Autodesk Inventor part; units mm, degrees
(part 2 of 2)
  spline S325 degree 2 poles (-2.5873, -27.7967) (-2.5873, -27.5088) (-2.9583, -27.0081) (-3.2851, -26.8732) knots 0 0 0 1 2 2 2
  spline S326 degree 2 poles (-3.2851, -26.8732) (-3.5393, -26.7669) (-3.9803, -26.7513) knots 0 0 0 1 1 1
  line L146 (-3.9803, -26.7513) -> (-3.3707, -25.5192)
  line L147 (-3.3707, -25.5192) -> (-2.232, -25.5192)
  line L148 (-1.433, -25.5192) -> (0.2686, -25.5192)
  line L149 (0.2686, -25.5192) -> (0.2686, -25.6074)
  line L150 (0.2686, -25.6074) -> (-0.7897, -28.759)
  line L151 (-0.7897, -28.759) -> (-1.0517, -28.759)
  line L152 (-1.0517, -28.759) -> (-0.1023, -25.9005)
  line L153 (-0.1023, -25.9005) -> (-0.9765, -25.9005)
  spline S327 degree 2 poles (-0.9765, -25.9005) (-1.2411, -25.9005) (-1.3526, -25.9628) knots 0 0 0 1 1 1
  spline S328 degree 2 poles (-1.3526, -25.9628) (-1.5498, -26.0717) (-1.6691, -26.2974) knots 0 0 0 1 1 1
  line L154 (-1.6691, -26.2974) -> (-1.7365, -26.2714)
  line L155 (-1.7365, -26.2714) -> (-1.433, -25.5192)
  spline S329 degree 2 poles (0.6577, -27.1248) (0.6577, -26.5827) (0.9845, -25.7993) (1.2569, -25.6074) knots 0 0 0 1 2 2 2
  spline S330 degree 2 poles (1.2569, -25.6074) (1.467, -25.4543) (1.6927, -25.4543) knots 0 0 0 1 1 1
  spline S331 degree 2 poles (1.6927, -25.4543) (2.0584, -25.4543) (2.3489, -25.8253) knots 0 0 0 1 1 1
  spline S332 degree 2 poles (2.3489, -25.8253) (2.7121, -26.287) (2.7121, -27.0756) knots 0 0 0 1 1 1
  spline S333 degree 2 poles (2.7121, -27.0756) (2.7121, -27.6281) (2.393, -28.4011) (1.9002, -28.7487) (1.6693, -28.7487) knots 0 0 0 1 2 3 3 3
  spline S334 degree 2 poles (1.6693, -28.7487) (1.2154, -28.7487) (0.9119, -28.2117) knots 0 0 0 1 1 1
  spline S335 degree 2 poles (0.9119, -28.2117) (0.6577, -27.7604) (0.6577, -27.1248) knots 0 0 0 1 1 1
  spline S336 degree 2 poles (1.1168, -27.1845) (1.1168, -27.8382) (1.2776, -28.2532) knots 0 0 0 1 1 1
  spline S337 degree 2 poles (1.2776, -28.2532) (1.4125, -28.6008) (1.6771, -28.6008) knots 0 0 0 1 1 1
  spline S338 degree 2 poles (1.6771, -28.6008) (1.8042, -28.6008) (2.074, -28.3751) (2.144, -28.108) knots 0 0 0 1 2 2 2
  spline S339 degree 2 poles (2.144, -28.108) (2.253, -27.7059) (2.253, -26.9744) knots 0 0 0 1 1 1
  spline S340 degree 2 poles (2.253, -26.9744) (2.253, -26.4297) (2.1414, -26.0691) knots 0 0 0 1 1 1
  spline S341 degree 2 poles (2.1414, -26.0691) (2.0558, -25.7993) (1.9235, -25.6878) knots 0 0 0 1 1 1
  spline S342 degree 2 poles (1.9235, -25.6878) (1.8276, -25.61) (1.6901, -25.61) knots 0 0 0 1 1 1
  spline S343 degree 2 poles (1.6901, -25.61) (1.5318, -25.61) (1.4073, -25.7526) knots 0 0 0 1 1 1
  spline S344 degree 2 poles (1.4073, -25.7526) (1.2387, -25.9472) (1.1168, -26.7798) (1.1168, -27.1845) knots 0 0 0 1 2 2 2
  spline S345 degree 2 poles (3.0571, -27.1248) (3.0571, -26.5827) (3.3839, -25.7993) (3.6563, -25.6074) knots 0 0 0 1 2 2 2
  spline S346 degree 2 poles (3.6563, -25.6074) (3.8664, -25.4543) (4.0921, -25.4543) knots 0 0 0 1 1 1
  spline S347 degree 2 poles (4.0921, -25.4543) (4.4578, -25.4543) (4.7484, -25.8253) knots 0 0 0 1 1 1
  spline S348 degree 2 poles (4.7484, -25.8253) (5.1115, -26.287) (5.1115, -27.0756) knots 0 0 0 1 1 1
  spline S349 degree 2 poles (5.1115, -27.0756) (5.1115, -27.6281) (4.7925, -28.4011) (4.2996, -28.7487) (4.0687, -28.7487) knots 0 0 0 1 2 3 3 3
  spline S350 degree 2 poles (4.0687, -28.7487) (3.6148, -28.7487) (3.3113, -28.2117) knots 0 0 0 1 1 1
  spline S351 degree 2 poles (3.3113, -28.2117) (3.0571, -27.7604) (3.0571, -27.1248) knots 0 0 0 1 1 1
  spline S352 degree 2 poles (3.5162, -27.1845) (3.5162, -27.8382) (3.677, -28.2532) knots 0 0 0 1 1 1
  spline S353 degree 2 poles (3.677, -28.2532) (3.8119, -28.6008) (4.0765, -28.6008) knots 0 0 0 1 1 1
  spline S354 degree 2 poles (4.0765, -28.6008) (4.2036, -28.6008) (4.4734, -28.3751) (4.5434, -28.108) knots 0 0 0 1 2 2 2
  spline S355 degree 2 poles (4.5434, -28.108) (4.6524, -27.7059) (4.6524, -26.9744) knots 0 0 0 1 1 1
  spline S356 degree 2 poles (4.6524, -26.9744) (4.6524, -26.4297) (4.5408, -26.0691) knots 0 0 0 1 1 1
  spline S357 degree 2 poles (4.5408, -26.0691) (4.4552, -25.7993) (4.3229, -25.6878) knots 0 0 0 1 1 1
  spline S358 degree 2 poles (4.3229, -25.6878) (4.227, -25.61) (4.0895, -25.61) knots 0 0 0 1 1 1
  spline S359 degree 2 poles (4.0895, -25.61) (3.9313, -25.61) (3.8067, -25.7526) knots 0 0 0 1 1 1
  spline S360 degree 2 poles (3.8067, -25.7526) (3.6381, -25.9472) (3.5162, -26.7798) (3.5162, -27.1845) knots 0 0 0 1 2 2 2
  spline S361 degree 2 poles (5.4565, -27.1248) (5.4565, -26.5827) (5.7833, -25.7993) (6.0557, -25.6074) knots 0 0 0 1 2 2 2
  spline S362 degree 2 poles (6.0557, -25.6074) (6.2658, -25.4543) (6.4915, -25.4543) knots 0 0 0 1 1 1
  spline S363 degree 2 poles (6.4915, -25.4543) (6.8572, -25.4543) (7.1478, -25.8253) knots 0 0 0 1 1 1
  spline S364 degree 2 poles (7.1478, -25.8253) (7.5109, -26.287) (7.5109, -27.0756) knots 0 0 0 1 1 1
  spline S365 degree 2 poles (7.5109, -27.0756) (7.5109, -27.6281) (7.1919, -28.4011) (6.699, -28.7487) (6.4681, -28.7487) knots 0 0 0 1 2 3 3 3
  spline S366 degree 2 poles (6.4681, -28.7487) (6.0142, -28.7487) (5.7107, -28.2117) knots 0 0 0 1 1 1
  spline S367 degree 2 poles (5.7107, -28.2117) (5.4565, -27.7604) (5.4565, -27.1248) knots 0 0 0 1 1 1
  spline S368 degree 2 poles (5.9156, -27.1845) (5.9156, -27.8382) (6.0765, -28.2532) knots 0 0 0 1 1 1
  spline S369 degree 2 poles (6.0765, -28.2532) (6.2113, -28.6008) (6.4759, -28.6008) knots 0 0 0 1 1 1
  spline S370 degree 2 poles (6.4759, -28.6008) (6.603, -28.6008) (6.8728, -28.3751) (6.9428, -28.108) knots 0 0 0 1 2 2 2
  spline S371 degree 2 poles (6.9428, -28.108) (7.0518, -27.7059) (7.0518, -26.9744) knots 0 0 0 1 1 1
  spline S372 degree 2 poles (7.0518, -26.9744) (7.0518, -26.4297) (6.9402, -26.0691) knots 0 0 0 1 1 1
  spline S373 degree 2 poles (6.9402, -26.0691) (6.8546, -25.7993) (6.7224, -25.6878) knots 0 0 0 1 1 1
  spline S374 degree 2 poles (6.7224, -25.6878) (6.6264, -25.61) (6.4889, -25.61) knots 0 0 0 1 1 1
  spline S375 degree 2 poles (6.4889, -25.61) (6.3307, -25.61) (6.2062, -25.7526) knots 0 0 0 1 1 1
  spline S376 degree 2 poles (6.2062, -25.7526) (6.0375, -25.9472) (5.9156, -26.7798) (5.9156, -27.1845) knots 0 0 0 1 2 2 2
  line L156 (8.2424, -25.8305) -> (9.0154, -25.4543)
  line L157 (9.0154, -25.4543) -> (9.0932, -25.4543)
  line L158 (9.0932, -25.4543) -> (9.0932, -28.1339)
  spline S377 degree 2 poles (9.0932, -28.1339) (9.0932, -28.4011) (9.1373, -28.5334) (9.2774, -28.6034) (9.4927, -28.6086) knots 0 0 0 1 2 3 3 3
  line L159 (9.4927, -28.6086) -> (9.4927, -28.6942)
  line L160 (9.4927, -28.6942) -> (8.2995, -28.6942)
  line L161 (8.2995, -28.6942) -> (8.2995, -28.6086)
  spline S378 degree 2 poles (8.2995, -28.6086) (8.5252, -28.6034) (8.6548, -28.536) (8.7067, -28.4218) (8.7067, -28.1339) knots 0 0 0 1 2 3 3 3
  line L162 (8.7067, -28.1339) -> (8.7067, -26.4219)
  spline S379 degree 2 poles (8.7067, -26.4219) (8.7067, -26.0743) (8.6834, -25.9757) knots 0 0 0 1 1 1
  spline S380 degree 2 poles (8.6834, -25.9757) (8.6678, -25.9005) (8.5796, -25.8305) (8.52, -25.8305) knots 0 0 0 1 2 2 2
  spline S381 degree 2 poles (8.52, -25.8305) (8.4318, -25.8305) (8.2787, -25.9031) knots 0 0 0 1 1 1
  line L163 (8.2787, -25.9031) -> (8.2424, -25.8305)
  line L164 (-11.5767, -33.1063) -> (-11.7998, -33.7159)
  line L165 (-11.7998, -33.7159) -> (-13.6726, -33.7159)
  line L166 (-13.6726, -33.7159) -> (-13.6726, -33.6303)
  spline S382 degree 2 poles (-13.6726, -33.6303) (-12.8451, -32.8755) (-12.1707, -31.9209) (-12.1707, -31.524) knots 0 0 0 1 2 2 2
  spline S383 degree 2 poles (-12.1707, -31.524) (-12.1707, -31.2231) (-12.5416, -30.834) (-12.7985, -30.834) knots 0 0 0 1 2 2 2
  spline S384 degree 2 poles (-12.7985, -30.834) (-13.0345, -30.834) (-13.4054, -31.109) (-13.4962, -31.3736) knots 0 0 0 1 2 2 2
  line L167 (-13.4962, -31.3736) -> (-13.5818, -31.3736)
  spline S385 degree 2 poles (-13.5818, -31.3736) (-13.5222, -30.9404) (-13.0397, -30.4761) (-12.6765, -30.4761) knots 0 0 0 1 2 2 2
  spline S386 degree 2 poles (-12.6765, -30.4761) (-12.29, -30.4761) (-11.7712, -30.9715) (-11.7712, -31.3087) knots 0 0 0 1 2 2 2
  spline S387 degree 2 poles (-11.7712, -31.3087) (-11.7712, -31.55) (-11.8828, -31.7912) knots 0 0 0 1 1 1
  spline S388 degree 2 poles (-11.8828, -31.7912) (-12.0566, -32.1699) (-12.4457, -32.5953) knots 0 0 0 1 1 1
  spline S389 degree 2 poles (-12.4457, -32.5953) (-13.0293, -33.2308) (-13.1746, -33.3631) knots 0 0 0 1 1 1
  line L168 (-13.1746, -33.3631) -> (-12.3445, -33.3631)
  spline S390 degree 2 poles (-12.3445, -33.3631) (-12.0903, -33.3631) (-11.888, -33.3268) (-11.7246, -33.2101) (-11.6623, -33.1063) knots 0 0 0 1 2 3 3 3
  line L169 (-11.6623, -33.1063) -> (-11.5767, -33.1063)
  spline S391 degree 2 poles (-10.5988, -31.9624) (-10.2227, -31.5084) (-9.8803, -31.5084) knots 0 0 0 1 1 1
  spline S392 degree 2 poles (-9.8803, -31.5084) (-9.7065, -31.5084) (-9.4548, -31.6848) (-9.3796, -31.8846) knots 0 0 0 1 2 2 2
  spline S393 degree 2 poles (-9.3796, -31.8846) (-9.3277, -32.0246) (-9.3277, -32.3152) knots 0 0 0 1 1 1
  line L170 (-9.3277, -32.3152) -> (-9.3277, -33.2308)
  spline S394 degree 2 poles (-9.3277, -33.2308) (-9.3277, -33.4332) (-9.294, -33.5058) knots 0 0 0 1 1 1
  spline S395 degree 2 poles (-9.294, -33.5058) (-9.2681, -33.5655) (-9.1539, -33.6303) (-9.0009, -33.6303) knots 0 0 0 1 2 2 2
  line L171 (-9.0009, -33.6303) -> (-9.0009, -33.7159)
  line L172 (-9.0009, -33.7159) -> (-10.0644, -33.7159)
  line L173 (-10.0644, -33.7159) -> (-10.0644, -33.6303)
  line L174 (-10.0644, -33.6303) -> (-10.0203, -33.6303)
  spline S396 degree 2 poles (-10.0203, -33.6303) (-9.8699, -33.6303) (-9.7506, -33.5395) (-9.7272, -33.4513) knots 0 0 0 1 2 2 2
  spline S397 degree 2 poles (-9.7272, -33.4513) (-9.7168, -33.415) (-9.7168, -33.2308) knots 0 0 0 1 1 1
  line L175 (-9.7168, -33.2308) -> (-9.7168, -32.3541)
  spline S398 degree 2 poles (-9.7168, -32.3541) (-9.7168, -32.061) (-9.8673, -31.7964) (-10.0463, -31.7964) knots 0 0 0 1 2 2 2
  spline S399 degree 2 poles (-10.0463, -31.7964) (-10.3238, -31.7964) (-10.5988, -32.0999) knots 0 0 0 1 1 1
  line L176 (-10.5988, -32.0999) -> (-10.5988, -33.2308)
  spline S400 degree 2 poles (-10.5988, -33.2308) (-10.5988, -33.4487) (-10.5728, -33.5006) knots 0 0 0 1 1 1
  spline S401 degree 2 poles (-10.5728, -33.5006) (-10.5391, -33.568) (-10.425, -33.6303) (-10.2486, -33.6303) knots 0 0 0 1 2 2 2
  line L177 (-10.2486, -33.6303) -> (-10.2486, -33.7159)
  line L178 (-10.2486, -33.7159) -> (-11.3147, -33.7159)
  line L179 (-11.3147, -33.7159) -> (-11.3147, -33.6303)
  line L180 (-11.3147, -33.6303) -> (-11.268, -33.6303)
  spline S402 degree 2 poles (-11.268, -33.6303) (-11.102, -33.6303) (-10.9879, -33.4643) (-10.9879, -33.2308) knots 0 0 0 1 2 2 2
  line L181 (-10.9879, -33.2308) -> (-10.9879, -32.4345)
  spline S403 degree 2 poles (-10.9879, -32.4345) (-10.9879, -32.0506) (-11.0242, -31.882) (-11.0968, -31.8197) (-11.1565, -31.8197) knots 0 0 0 1 2 3 3 3
  spline S404 degree 2 poles (-11.1565, -31.8197) (-11.2213, -31.8197) (-11.3121, -31.856) knots 0 0 0 1 1 1
  line L182 (-11.3121, -31.856) -> (-11.3484, -31.7704)
  line L183 (-11.3484, -31.7704) -> (-10.6999, -31.5084)
  line L184 (-10.6999, -31.5084) -> (-10.5988, -31.5084)
  line L185 (-10.5988, -31.5084) -> (-10.5988, -31.9624)
  spline S405 degree 2 poles (-7.3148, -33.4747) (-7.4705, -33.6381) (-7.7714, -33.7808) (-7.9452, -33.7808) knots 0 0 0 1 2 2 2
  spline S406 degree 2 poles (-7.9452, -33.7808) (-8.2953, -33.7808) (-8.8193, -33.1945) (-8.8193, -32.7328) knots 0 0 0 1 2 2 2
  spline S407 degree 2 poles (-8.8193, -32.7328) (-8.8193, -32.2737) (-8.2383, -31.5084) (-7.7817, -31.5084) knots 0 0 0 1 2 2 2
  spline S408 degree 2 poles (-7.7817, -31.5084) (-7.499, -31.5084) (-7.3148, -31.69) knots 0 0 0 1 1 1
  line L186 (-7.3148, -31.69) -> (-7.3148, -31.288)
  spline S409 degree 2 poles (-7.3148, -31.288) (-7.3148, -30.9222) (-7.3511, -30.7562) (-7.4238, -30.6965) (-7.4808, -30.6965) knots 0 0 0 1 2 3 3 3
  spline S410 degree 2 poles (-7.4808, -30.6965) (-7.5405, -30.6965) (-7.6417, -30.7329) knots 0 0 0 1 1 1
  line L187 (-7.6417, -30.7329) -> (-7.6728, -30.6473)
  line L188 (-7.6728, -30.6473) -> (-7.0347, -30.3853)
  line L189 (-7.0347, -30.3853) -> (-6.9283, -30.3853)
  line L190 (-6.9283, -30.3853) -> (-6.9283, -32.8677)
  spline S411 degree 2 poles (-6.9283, -32.8677) (-6.9283, -33.2412) (-6.892, -33.4072) (-6.8168, -33.4721) (-6.7649, -33.4721) knots 0 0 0 1 2 3 3 3
  spline S412 degree 2 poles (-6.7649, -33.4721) (-6.7027, -33.4721) (-6.5963, -33.4332) knots 0 0 0 1 1 1
  line L191 (-6.5963, -33.4332) -> (-6.5704, -33.5188)
  line L192 (-6.5704, -33.5188) -> (-7.2059, -33.7808)
  line L193 (-7.2059, -33.7808) -> (-7.3148, -33.7808)
  line L194 (-7.3148, -33.7808) -> (-7.3148, -33.4747)
  line L195 (-7.3148, -33.3087) -> (-7.3148, -32.2088)
  spline S413 degree 2 poles (-7.3148, -32.2088) (-7.3278, -32.048) (-7.4705, -31.786) (-7.7013, -31.6537) (-7.8103, -31.6537) knots 0 0 0 1 2 3 3 3
  spline S414 degree 2 poles (-7.8103, -31.6537) (-8.0178, -31.6537) (-8.1786, -31.8379) knots 0 0 0 1 1 1
  spline S415 degree 2 poles (-8.1786, -31.8379) (-8.3913, -32.0817) (-8.3913, -32.5486) knots 0 0 0 1 1 1
  spline S416 degree 2 poles (-8.3913, -32.5486) (-8.3913, -33.0207) (-7.9789, -33.5239) (-7.7273, -33.5239) knots 0 0 0 1 2 2 2
  spline S417 degree 2 poles (-7.7273, -33.5239) (-7.5146, -33.5239) (-7.3148, -33.3087) knots 0 0 0 1 1 1
  line L196 (-3.1749, -30.4683) -> (-3.1749, -31.5655)
  line L197 (-3.1749, -31.5655) -> (-3.2605, -31.5655)
  spline S418 degree 2 poles (-3.2605, -31.5655) (-3.302, -31.2491) (-3.5225, -30.8755) (-3.9245, -30.655) (-4.1424, -30.655) knots 0 0 0 1 2 3 3 3
  spline S419 degree 2 poles (-4.1424, -30.655) (-4.3863, -30.655) (-4.7053, -30.9533) (-4.7053, -31.1427) knots 0 0 0 1 2 2 2
  spline S420 degree 2 poles (-4.7053, -31.1427) (-4.7053, -31.288) (-4.6041, -31.4073) knots 0 0 0 1 1 1
  spline S421 degree 2 poles (-4.6041, -31.4073) (-4.4589, -31.5837) (-3.9116, -31.8768) knots 0 0 0 1 1 1
  spline S422 degree 2 poles (-3.9116, -31.8768) (-3.468, -32.1154) (-3.1412, -32.3696) (-2.9648, -32.7172) (-2.9648, -32.9066) knots 0 0 0 1 2 3 3 3
  spline S423 degree 2 poles (-2.9648, -32.9066) (-2.9648, -33.2671) (-3.5251, -33.7885) (-3.966, -33.7885) knots 0 0 0 1 2 2 2
  spline S424 degree 2 poles (-3.966, -33.7885) (-4.1035, -33.7885) (-4.2254, -33.7678) knots 0 0 0 1 1 1
  spline S425 degree 2 poles (-4.2254, -33.7678) (-4.2981, -33.7548) (-4.7546, -33.607) (-4.8169, -33.607) knots 0 0 0 1 2 2 2
  spline S426 degree 2 poles (-4.8169, -33.607) (-4.8739, -33.607) (-4.944, -33.677) (-4.9595, -33.7885) knots 0 0 0 1 2 2 2
  line L198 (-4.9595, -33.7885) -> (-5.0451, -33.7885)
  line L199 (-5.0451, -33.7885) -> (-5.0451, -32.6991)
  line L200 (-5.0451, -32.6991) -> (-4.9595, -32.6991)
  spline S427 degree 2 poles (-4.9595, -32.6991) (-4.8999, -33.0415) (-4.6923, -33.3813) (-4.2669, -33.607) (-4.0153, -33.607) knots 0 0 0 1 2 3 3 3
  spline S428 degree 2 poles (-4.0153, -33.607) (-3.7222, -33.607) (-3.3824, -33.2983) (-3.3824, -33.0856) knots 0 0 0 1 2 2 2
  spline S429 degree 2 poles (-3.3824, -33.0856) (-3.3824, -32.9688) (-3.5121, -32.7302) (-3.647, -32.6264) knots 0 0 0 1 2 2 2
  spline S430 degree 2 poles (-3.647, -32.6264) (-3.7378, -32.5564) (-4.5549, -32.0999) (-4.8999, -31.8275) (-5.0788, -31.5007) (-5.0788, -31.3035) knots 0 0 0 1 2 3 4 4 4
  spline S431 degree 2 poles (-5.0788, -31.3035) (-5.0788, -30.9611) (-4.5523, -30.4683) (-4.145, -30.4683) knots 0 0 0 1 2 2 2
  spline S432 degree 2 poles (-4.145, -30.4683) (-3.8934, -30.4683) (-3.6081, -30.5928) knots 0 0 0 1 1 1
  spline S433 degree 2 poles (-3.6081, -30.5928) (-3.4758, -30.6498) (-3.4213, -30.6498) knots 0 0 0 1 1 1
  spline S434 degree 2 poles (-3.4213, -30.6498) (-3.3616, -30.6498) (-3.2838, -30.5772) (-3.2605, -30.4683) knots 0 0 0 1 2 2 2
  line L201 (-3.2605, -30.4683) -> (-3.1749, -30.4683)
  spline S435 degree 2 poles (-2.2021, -32.38) (-2.2047, -32.8573) (-1.9713, -33.1271) knots 0 0 0 1 1 1
  spline S436 degree 2 poles (-1.9713, -33.1271) (-1.7352, -33.3994) (-1.4188, -33.3994) knots 0 0 0 1 1 1
  spline S437 degree 2 poles (-1.4188, -33.3994) (-1.2087, -33.3994) (-0.8974, -33.1686) (-0.791, -32.8858) knots 0 0 0 1 2 2 2
  line L202 (-0.791, -32.8858) -> (-0.7184, -32.9325)
  spline S438 degree 2 poles (-0.7184, -32.9325) (-0.7677, -33.2542) (-1.2398, -33.7808) (-1.5978, -33.7808) knots 0 0 0 1 2 2 2
  spline S439 degree 2 poles (-1.5978, -33.7808) (-1.9843, -33.7808) (-2.5342, -33.179) (-2.5342, -32.6731) knots 0 0 0 1 2 2 2
  spline S440 degree 2 poles (-2.5342, -32.6731) (-2.5342, -32.1232) (-1.9687, -31.5084) (-1.5433, -31.5084) knots 0 0 0 1 2 2 2
  spline S441 degree 2 poles (-1.5433, -31.5084) (-1.1827, -31.5084) (-0.7184, -31.9831) (-0.7184, -32.38) knots 0 0 0 1 2 2 2
  line L203 (-0.7184, -32.38) -> (-2.2021, -32.38)
  line L204 (-2.2021, -32.2451) -> (-1.2061, -32.2451)
  spline S442 degree 2 poles (-1.2061, -32.2451) (-1.219, -32.0402) (-1.2554, -31.9546) knots 0 0 0 1 1 1
  spline S443 degree 2 poles (-1.2554, -31.9546) (-1.315, -31.8249) (-1.5459, -31.6745) (-1.673, -31.6745) knots 0 0 0 1 2 2 2
  spline S444 degree 2 poles (-1.673, -31.6745) (-1.8675, -31.6745) (-2.1762, -31.9754) (-2.2021, -32.2451) knots 0 0 0 1 2 2 2
  line L205 (-0.5887, -31.7834) -> (0.0728, -31.5162)
  line L206 (0.0728, -31.5162) -> (0.1609, -31.5162)
  line L207 (0.1609, -31.5162) -> (0.1609, -32.0195)
  spline S445 degree 2 poles (0.1609, -32.0195) (0.327, -31.7367) (0.6616, -31.5084) (0.8457, -31.5084) knots 0 0 0 1 2 2 2
  spline S446 degree 2 poles (0.8457, -31.5084) (1.17, -31.5084) (1.3853, -31.7601) knots 0 0 0 1 1 1
  spline S447 degree 2 poles (1.3853, -31.7601) (1.6499, -32.0713) (1.6499, -32.5668) knots 0 0 0 1 1 1
  spline S448 degree 2 poles (1.6499, -32.5668) (1.6499, -33.1219) (1.3308, -33.4824) knots 0 0 0 1 1 1
  spline S449 degree 2 poles (1.3308, -33.4824) (1.0688, -33.7808) (0.672, -33.7808) knots 0 0 0 1 1 1
  spline S450 degree 2 poles (0.672, -33.7808) (0.4982, -33.7808) (0.3711, -33.7315) knots 0 0 0 1 1 1
  spline S451 degree 2 poles (0.3711, -33.7315) (0.2777, -33.6977) (0.1609, -33.5914) knots 0 0 0 1 1 1
  line L208 (0.1609, -33.5914) -> (0.1609, -34.2451)
  spline S452 degree 2 poles (0.1609, -34.2451) (0.1609, -34.4656) (0.2154, -34.5849) (0.3477, -34.6549) (0.5241, -34.6549) knots 0 0 0 1 2 3 3 3
  line L209 (0.5241, -34.6549) -> (0.5241, -34.7405)
  line L210 (0.5241, -34.7405) -> (-0.6017, -34.7405)
  line L211 (-0.6017, -34.7405) -> (-0.6017, -34.6549)
  line L212 (-0.6017, -34.6549) -> (-0.542, -34.6549)
  spline S453 degree 2 poles (-0.542, -34.6549) (-0.4149, -34.6575) (-0.3215, -34.6056) knots 0 0 0 1 1 1
  spline S454 degree 2 poles (-0.3215, -34.6056) (-0.2774, -34.5797) (-0.2281, -34.4656) (-0.2281, -34.2295) knots 0 0 0 1 2 2 2
  line L213 (-0.2281, -34.2295) -> (-0.2281, -32.2036)
  spline S455 degree 2 poles (-0.2281, -32.2036) (-0.2281, -31.9935) (-0.2645, -31.882) (-0.3475, -31.8249) (-0.4175, -31.8249) knots 0 0 0 1 2 3 3 3
  spline S456 degree 2 poles (-0.4175, -31.8249) (-0.4746, -31.8249) (-0.5602, -31.8586) knots 0 0 0 1 1 1
  line L214 (-0.5602, -31.8586) -> (-0.5887, -31.7834)
  line L215 (0.1609, -32.1569) -> (0.1609, -32.9585)
  spline S457 degree 2 poles (0.1609, -32.9585) (0.1609, -33.2179) (0.1817, -33.2983) knots 0 0 0 1 1 1
  spline S458 degree 2 poles (0.1817, -33.2983) (0.2154, -33.4358) (0.4696, -33.6407) (0.6642, -33.6407) knots 0 0 0 1 2 2 2
  spline S459 degree 2 poles (0.6642, -33.6407) (0.8976, -33.6407) (1.0429, -33.4591) knots 0 0 0 1 1 1
  spline S460 degree 2 poles (1.0429, -33.4591) (1.2322, -33.2205) (1.2322, -32.7873) knots 0 0 0 1 1 1
  spline S461 degree 2 poles (1.2322, -32.7873) (1.2322, -32.2944) (1.0169, -32.0298) knots 0 0 0 1 1 1
  spline S462 degree 2 poles (1.0169, -32.0298) (0.8665, -31.8483) (0.6616, -31.8483) knots 0 0 0 1 1 1
  spline S463 degree 2 poles (0.6616, -31.8483) (0.55, -31.8483) (0.4385, -31.9053) knots 0 0 0 1 1 1
  spline S464 degree 2 poles (0.4385, -31.9053) (0.3555, -31.9468) (0.1609, -32.1569) knots 0 0 0 1 1 1
  line L216 (2.5915, -30.8651) -> (2.5915, -31.5707)
  line L217 (2.5915, -31.5707) -> (3.0921, -31.5707)
  line L218 (3.0921, -31.5707) -> (3.0921, -31.7341)
  line L219 (3.0921, -31.7341) -> (2.5915, -31.7341)
  line L220 (2.5915, -31.7341) -> (2.5915, -33.1271)
  spline S465 degree 2 poles (2.5915, -33.1271) (2.5915, -33.3346) (2.7108, -33.4799) (2.8042, -33.4799) knots 0 0 0 1 2 2 2
  spline S466 degree 2 poles (2.8042, -33.4799) (2.882, -33.4799) (3.0299, -33.3839) (3.0688, -33.2905) knots 0 0 0 1 2 2 2
  line L221 (3.0688, -33.2905) -> (3.1596, -33.2905)
  spline S467 degree 2 poles (3.1596, -33.2905) (3.0765, -33.5214) (2.7757, -33.7522) (2.6174, -33.7522) knots 0 0 0 1 2 2 2
  spline S468 degree 2 poles (2.6174, -33.7522) (2.5085, -33.7522) (2.301, -33.6329) (2.2024, -33.4098) (2.2024, -33.179) knots 0 0 0 1 2 3 3 3
  line L222 (2.2024, -33.179) -> (2.2024, -31.7341)
  line L223 (2.2024, -31.7341) -> (1.8626, -31.7341)
  line L224 (1.8626, -31.7341) -> (1.8626, -31.6563)
  spline S469 degree 2 poles (1.8626, -31.6563) (1.9923, -31.6044) (2.262, -31.3606) (2.3684, -31.192) knots 0 0 0 1 2 2 2
  spline S470 degree 2 poles (2.3684, -31.192) (2.4229, -31.1012) (2.5188, -30.8651) knots 0 0 0 1 1 1
  line L225 (2.5188, -30.8651) -> (2.5915, -30.8651)
  line L226 (6.5473, -33.1063) -> (6.3242, -33.7159)
  line L227 (6.3242, -33.7159) -> (4.4513, -33.7159)
  line L228 (4.4513, -33.7159) -> (4.4513, -33.6303)
  spline S471 degree 2 poles (4.4513, -33.6303) (5.2788, -32.8755) (5.9532, -31.9209) (5.9532, -31.524) knots 0 0 0 1 2 2 2
  spline S472 degree 2 poles (5.9532, -31.524) (5.9532, -31.2231) (5.5823, -30.834) (5.3255, -30.834) knots 0 0 0 1 2 2 2
  spline S473 degree 2 poles (5.3255, -30.834) (5.0895, -30.834) (4.7185, -31.109) (4.6277, -31.3736) knots 0 0 0 1 2 2 2
  line L229 (4.6277, -31.3736) -> (4.5421, -31.3736)
  spline S474 degree 2 poles (4.5421, -31.3736) (4.6018, -30.9404) (5.0843, -30.4761) (5.4474, -30.4761) knots 0 0 0 1 2 2 2
  spline S475 degree 2 poles (5.4474, -30.4761) (5.8339, -30.4761) (6.3527, -30.9715) (6.3527, -31.3087) knots 0 0 0 1 2 2 2
  spline S476 degree 2 poles (6.3527, -31.3087) (6.3527, -31.55) (6.2412, -31.7912) knots 0 0 0 1 1 1
  spline S477 degree 2 poles (6.2412, -31.7912) (6.0674, -32.1699) (5.6783, -32.5953) knots 0 0 0 1 1 1
  spline S478 degree 2 poles (5.6783, -32.5953) (5.0946, -33.2308) (4.9494, -33.3631) knots 0 0 0 1 1 1
  line L230 (4.9494, -33.3631) -> (5.7794, -33.3631)
  spline S479 degree 2 poles (5.7794, -33.3631) (6.0337, -33.3631) (6.236, -33.3268) (6.3994, -33.2101) (6.4617, -33.1063) knots 0 0 0 1 2 3 3 3
  line L231 (6.4617, -33.1063) -> (6.5473, -33.1063)
  spline S480 degree 2 poles (6.9208, -32.1466) (6.9208, -31.6044) (7.2476, -30.821) (7.52, -30.6291) knots 0 0 0 1 2 2 2
  spline S481 degree 2 poles (7.52, -30.6291) (7.7301, -30.4761) (7.9558, -30.4761) knots 0 0 0 1 1 1
  spline S482 degree 2 poles (7.9558, -30.4761) (8.3215, -30.4761) (8.612, -30.847) knots 0 0 0 1 1 1
  spline S483 degree 2 poles (8.612, -30.847) (8.9752, -31.3087) (8.9752, -32.0973) knots 0 0 0 1 1 1
  spline S484 degree 2 poles (8.9752, -32.0973) (8.9752, -32.6498) (8.6561, -33.4228) (8.1633, -33.7704) (7.9324, -33.7704) knots 0 0 0 1 2 3 3 3
  spline S485 degree 2 poles (7.9324, -33.7704) (7.4785, -33.7704) (7.175, -33.2334) knots 0 0 0 1 1 1
  spline S486 degree 2 poles (7.175, -33.2334) (6.9208, -32.7821) (6.9208, -32.1466) knots 0 0 0 1 1 1
  spline S487 degree 2 poles (7.3799, -32.2062) (7.3799, -32.8599) (7.5407, -33.2749) knots 0 0 0 1 1 1
  spline S488 degree 2 poles (7.5407, -33.2749) (7.6756, -33.6225) (7.9402, -33.6225) knots 0 0 0 1 1 1
  spline S489 degree 2 poles (7.9402, -33.6225) (8.0673, -33.6225) (8.3371, -33.3968) (8.4071, -33.1297) knots 0 0 0 1 2 2 2
  spline S490 degree 2 poles (8.4071, -33.1297) (8.5161, -32.7276) (8.5161, -31.9961) knots 0 0 0 1 1 1
  spline S491 degree 2 poles (8.5161, -31.9961) (8.5161, -31.4514) (8.4045, -31.0908) knots 0 0 0 1 1 1
  spline S492 degree 2 poles (8.4045, -31.0908) (8.3189, -30.821) (8.1866, -30.7095) knots 0 0 0 1 1 1
  spline S493 degree 2 poles (8.1866, -30.7095) (8.0907, -30.6317) (7.9532, -30.6317) knots 0 0 0 1 1 1
  spline S494 degree 2 poles (7.9532, -30.6317) (7.795, -30.6317) (7.6704, -30.7744) knots 0 0 0 1 1 1
  spline S495 degree 2 poles (7.6704, -30.7744) (7.5018, -30.9689) (7.3799, -31.8016) (7.3799, -32.2062) knots 0 0 0 1 2 2 2
  line L232 (11.3461, -33.1063) -> (11.123, -33.7159)
  line L233 (11.123, -33.7159) -> (9.2502, -33.7159)
  line L234 (9.2502, -33.7159) -> (9.2502, -33.6303)
  spline S496 degree 2 poles (9.2502, -33.6303) (10.0776, -32.8755) (10.7521, -31.9209) (10.7521, -31.524) knots 0 0 0 1 2 2 2
  spline S497 degree 2 poles (10.7521, -31.524) (10.7521, -31.2231) (10.3811, -30.834) (10.1243, -30.834) knots 0 0 0 1 2 2 2
  spline S498 degree 2 poles (10.1243, -30.834) (9.8883, -30.834) (9.5173, -31.109) (9.4265, -31.3736) knots 0 0 0 1 2 2 2
  line L235 (9.4265, -31.3736) -> (9.3409, -31.3736)
  spline S499 degree 2 poles (9.3409, -31.3736) (9.4006, -30.9404) (9.8831, -30.4761) (10.2462, -30.4761) knots 0 0 0 1 2 2 2
  spline S500 degree 2 poles (10.2462, -30.4761) (10.6327, -30.4761) (11.1515, -30.9715) (11.1515, -31.3087) knots 0 0 0 1 2 2 2
  spline S501 degree 2 poles (11.1515, -31.3087) (11.1515, -31.55) (11.04, -31.7912) knots 0 0 0 1 1 1
  spline S502 degree 2 poles (11.04, -31.7912) (10.8662, -32.1699) (10.4771, -32.5953) knots 0 0 0 1 1 1
  spline S503 degree 2 poles (10.4771, -32.5953) (9.8935, -33.2308) (9.7482, -33.3631) knots 0 0 0 1 1 1
  line L236 (9.7482, -33.3631) -> (10.5783, -33.3631)
  spline S504 degree 2 poles (10.5783, -33.3631) (10.8325, -33.3631) (11.0348, -33.3268) (11.1982, -33.2101) (11.2605, -33.1063) knots 0 0 0 1 2 3 3 3
  line L237 (11.2605, -33.1063) -> (11.3461, -33.1063)
  line L238 (13.6288, -30.5409) -> (13.4472, -30.9378)
  line L239 (13.4472, -30.9378) -> (12.4926, -30.9378)
  line L240 (12.4926, -30.9378) -> (12.2825, -31.3632)
  spline S505 degree 2 poles (12.2825, -31.3632) (12.9024, -31.454) (13.2656, -31.8249) knots 0 0 0 1 1 1
  spline S506 degree 2 poles (13.2656, -31.8249) (13.5769, -32.144) (13.5769, -32.5746) knots 0 0 0 1 1 1
  spline S507 degree 2 poles (13.5769, -32.5746) (13.5769, -32.8236) (13.372, -33.2516) (13.0633, -33.5499) (12.8739, -33.6407) knots 0 0 0 1 2 3 3 3
  spline S508 degree 2 poles (12.8739, -33.6407) (12.6041, -33.7704) (12.3214, -33.7704) knots 0 0 0 1 1 1
  spline S509 degree 2 poles (12.3214, -33.7704) (12.0335, -33.7704) (11.7741, -33.5758) (11.7741, -33.4591) knots 0 0 0 1 2 2 2
  spline S510 degree 2 poles (11.7741, -33.4591) (11.7741, -33.3943) (11.8804, -33.2931) (11.9634, -33.2931) knots 0 0 0 1 2 2 2
  spline S511 degree 2 poles (11.9634, -33.2931) (12.0231, -33.2931) (12.1165, -33.332) (12.2254, -33.4098) knots 0 0 0 1 2 2 2
  spline S512 degree 2 poles (12.2254, -33.4098) (12.4018, -33.5291) (12.5834, -33.5317) knots 0 0 0 1 1 1
  spline S513 degree 2 poles (12.5834, -33.5317) (12.8558, -33.5317) (13.2734, -33.1167) (13.2734, -32.8184) knots 0 0 0 1 2 2 2
  spline S514 degree 2 poles (13.2734, -32.8184) (13.2734, -32.5305) (12.9024, -32.0298) (12.5756, -31.8949) knots 0 0 0 1 2 2 2
  spline S515 degree 2 poles (12.5756, -31.8949) (12.3214, -31.7886) (11.8804, -31.773) knots 0 0 0 1 1 1
  line L241 (11.8804, -31.773) -> (12.49, -30.5409)
  line L242 (12.49, -30.5409) -> (13.6288, -30.5409)
  point P0 (25.4, -19.05)
  dimension "d0" = 53.086
  dimension "d1" = 50.8
  constraints: 4 other
emboss "Emboss1" sketch "Sketch8" operation cut depth 2 direction (0, 0, 1)
body "Solid1"
